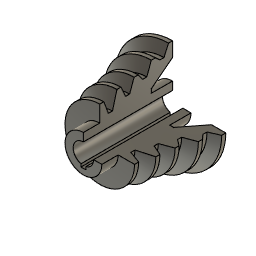
Sketch24_Final v0 (Autodesk Fusion 360 design; units mm, degrees)
Autodesk Fusion 360 part; units mm, degrees
sketch "Sketch1" plane through (0, 0, 0) normal (0, 0, 1) x (1, 0, 0)
  line L0 (12.5, 0) -> (22.5, 0)
  line L1 (12.5, 0) -> (12.5, 20)
  line L2 (22.5, 0) -> (22.5, 20)
  line L3 (22.5, 20) -> (42.5, 20)
  line L4 (42.5, 20) -> (42.5, 25)
  line L5 (42.5, 25) -> (22.5, 25)
  line L6 (0, 0) -> (0, 115)
  line L7 (0, 25) -> (0, 41)
  line L8 (22.5, 41) -> (47.5, 41)
  line L9 (47.5, 41) -> (47.5, 46)
  line L10 (47.5, 46) -> (22.5, 46)
  line L11 (0, 46) -> (0, 62)
  line L12 (22.5, 62) -> (50, 62)
  line L13 (50, 62) -> (50, 67)
  line L14 (50, 67) -> (22.5, 67)
  line L15 (0, 67) -> (0, 83)
  line L16 (57.5, 83) -> (57.5, 88)
  line L17 (0, 88) -> (0, 104)
  line L18 (65, 104) -> (65, 109)
  line L19 (52.5, 98.5) -> (52.5, 93.5)
  line L20 (65, 104) -> (52.5, 98.5)
  line L21 (52.5, 93.5) -> (57.5, 88)
  line L22 (12.5, 20) -> (12.5, 109)
  line L23 (22.5, 20) -> (22.5, 109)
  line L24 (0, 83) -> (0, 77.5)
  line L25 (23, 77.5) -> (42.5, 77.5)
  line L26 (42.5, 77.5) -> (42.5, 72.5)
  line L27 (42.5, 72.5) -> (22.5, 72.5041)
  line L28 (42.5, 77.5) -> (57.5, 83)
  line L29 (42.5, 72.5) -> (50, 67)
  line L30 (0, 62) -> (0, 56.5)
  line L31 (22.5, 56.5) -> (35, 56.5)
  line L32 (35, 56.5) -> (35, 51.5)
  line L33 (35, 56.5) -> (50, 62)
  line L34 (35, 51.5) -> (47.5, 46)
  line L35 (0, 41) -> (0, 35.5)
  line L36 (22.5, 35.5) -> (27.5, 35.5)
  line L37 (27.5, 35.5) -> (27.5, 30.5)
  line L38 (47.5, 41) -> (27.5, 35.5)
  line L39 (27.5, 30.5) -> (42.5, 25)
  line L40 (0, 93.5) -> (-0.0024, 93.5)
  line L41 (35, 51.5) -> (22.5, 51.5)
  line L42 (0, 51.5) -> (-0.0011, 51.5)
  line L43 (27.5, 30.5) -> (22.5, 30.5)
  line L44 (0, 30.5) -> (-0.1134, 30.5)
  line L45 (12.5, 109) -> (12.5, 64)
  line L46 (22.5, 76.8571) -> (47.5, 109)
  line L47 (43.6111, 104) -> (65, 104)
  line L48 (39.3333, 98.5) -> (52.5, 98.5)
  line L49 (52.5, 93.5) -> (35.4444, 93.5)
  line L50 (57.5, 88) -> (31.1667, 88)
  line L51 (27.2778, 83) -> (57.5, 83)
  line L52 (65, 109) -> (47.5, 109)
  line L53 (22.5, 109) -> (12.5, 109)
  line L54 (27.2778, 83) -> (22.5, 83)
  dimension "d1" = 12.5
  dimension "d2" = 22.5
  dimension "d3" = 20
  dimension "d6" = 5
  dimension "d7" = 115
  dimension "d8" = 16
  dimension "d9" = 47.5
  dimension "d10" = 5
  dimension "d11" = 16
  dimension "d12" = 50
  dimension "d13" = 5
  dimension "d14" = 16
  dimension "d15" = 57.5
  dimension "d16" = 5
  dimension "d17" = 16
  dimension "d18" = 65
  dimension "d19" = 5
  dimension "d24" = 5
  dimension "d25" = 90
  dimension "d26" = 5.5
  dimension "d27" = 42.5
  dimension "d28" = 5
  dimension "d29" = 5.5
  dimension "d30" = 35
  dimension "d31" = 5
  dimension "d32" = 90
  dimension "d33" = 5.5
  dimension "d34" = 27.5
  dimension "d35" = 5
  dimension "d36" = 90
  dimension "d37" = 45
  dimension "d38" = 25
  constraint perpendicular L0 L1
  constraint perpendicular L0 L2
  constraint perpendicular L2 L3
  constraint perpendicular L3 L4
  constraint perpendicular L4 L5
  constraint coincident L6.start origin
  constraint perpendicular L5 L7
  constraint perpendicular L7 L8
  constraint perpendicular L8 L9
  constraint coincident L6 L11.start
  constraint perpendicular L6 L10
  constraint perpendicular L10 L11
  constraint perpendicular L6 L12
  constraint perpendicular L12 L13
  constraint coincident L6 L15.start
  constraint perpendicular L6 L14
  constraint perpendicular L14 L15
  constraint coincident L6 L17.start
  constraint perpendicular L6 L50
  constraint perpendicular L17 L50
  constraint perpendicular L18 L50
  constraint perpendicular L6 L52
  constraint perpendicular L17 L49
  constraint perpendicular L22 L52
  constraint coincident L23.end L52
  constraint perpendicular L23 L52
  constraint perpendicular L15 L25
  constraint perpendicular L25 L26
  constraint perpendicular L12 L30
  constraint perpendicular L22 L31
  constraint perpendicular L31 L32
  constraint perpendicular L8 L35
  constraint perpendicular L23 L36
  constraint perpendicular L36 L37
  constraint coincident L6 L40.start
  constraint collinear L40 L49
  constraint coincident L6 L42.start
  constraint collinear L41 L42
  constraint coincident L6 L44.start
  constraint collinear L43 L44
  constraint perpendicular L25 L45
  constraint coincident L46 L47.start
  constraint coincident L46 L48.start
  constraint coincident L46 L49.end
  constraint coincident L46 L50.end
  constraint coincident L46 L51.start
  constraint collinear L52 L53
  constraint coincident L23 L27.end
  constraint coincident L23 L14.end
  constraint coincident L23 L12.start
  constraint coincident L23 L46.start
  constraint coincident L23 L31.start
  constraint coincident L23 L41.end
  constraint coincident L23 L10.end
  constraint coincident L23 L8.start
  constraint coincident L23 L36.start
  constraint coincident L23 L43.end
  constraint coincident L23 L5.end
  constraint perpendicular L23 L54
  constraint coincident L23 L54.end
  constraint coincident L46 L25.start
  measures "d1" distance of L6.start L0.start
  measures "d2" distance of L6.start L0.end
  measures "d3" distance of L0.start L1.end
  measures "d6" distance of L3.end L4.end
  measures "d7" distance of L6.start L6.end
  measures "d8" distance of L7.start L7.end
  measures "d9" distance of L7.end L8.end
  measures "d10" distance of L8.end L9.end
  measures "d11" distance of L11.start L11.end
  measures "d12" distance of L11.end L12.end
  measures "d13" distance of L12.end L13.end
  measures "d14" distance of L15.start L15.end
  measures "d15" distance of L15.end L16.start
  measures "d16" distance of L16.start L16.end
  measures "d17" distance of L17.start L17.end
  measures "d18" distance of L17.end L18.start
  measures "d19" distance of L18.start L18.end
  measures "d24" distance of L19.start L19.end
  measures "d25" angle of L19 L49
  measures "d26" distance of L15.end L24.end
  measures "d27" distance of L24.end L25.end
  measures "d28" distance of L25.end L26.end
  measures "d29" distance of L11.end L30.end
  measures "d30" distance of L30.end L31.end
  measures "d31" distance of L31.end L32.end
  measures "d32" angle of L32 L41
  measures "d33" distance of L7.end L35.end
  measures "d34" distance of L35.end L36.end
  measures "d35" distance of L36.end L37.end
  measures "d36" angle of L37 L43
  measures "d37" distance of L22.end L45.end
  measures "d38" distance of L23.end L46.end
revolve "Revolve1" add sketch "Sketch1" angle 360 about axis through (0, 0, 0) along (0, 1, 0)
sketch "Sketch2" plane through (0, 0, 0) normal (0, 1, 0) x (1, 0, 0)
  line L0 (0, 12.5) -> (0, 15.5)
  line L1 (0, 15.5) -> (3, 15.5)
  line L2 (3, 15.5) -> (-3, 15.5)
  line L3 (-3, 15.5) -> (-3, 12)
  line L4 (-3, 12) -> (3, 12)
  line L5 (3, 12) -> (3, 15.5)
  dimension "d40" = 3
  dimension "d41" = 6
  constraint vertical L0
  constraint perpendicular L0 L1
  constraint perpendicular L0 L2
  constraint perpendicular L2 L3
  constraint perpendicular L3 L4
  constraint perpendicular L1 L5
  measures "d40" distance of L0.start L0.end
  measures "d41" distance of L1.end L2.end
extrude "Extrude1" cut sketch "Sketch2" along normal blind 115
sketch "Sketch3" plane through (0, 0, 0) normal (0, 1, 0) x (1, 0, 0)
  line L0 (0, -90) -> (100, -90)
  line L1 (100, -90) -> (100, 0)
  line L2 (100, 0) -> (0, 0)
  line L3 (0, 0) -> (0, -90)
  constraint horizontal L0
  constraint vertical L1
  constraint horizontal L2
  constraint vertical L3
extrude "Extrude2" cut sketch "Sketch3" along normal blind 115
